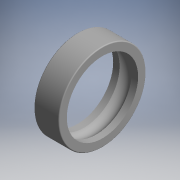
# Autodesk Inventor part: 6001JRX Outer Ring
Saved by Autodesk Inventor 2017.3 (Build 213256000, 256)
## iProperties
Part Number: 6001JRX Outer Ring
Material: Generic
Catalog Web Link: www.cadenas.de
Description: Open type or-Deep Groove Ball Bearings
Vendor: NTN
Document SubType Name: Modeling
Designer: partserver
Manufacturer: NTN
Mass: 1.44189 g
Surface Area: 17.2678 cm^2
Volume: 1.44189 cm^3
Density: 1 g/cm^3
Appearance: PSOLRGB-192-192-192
Category: PARTsolutions
Company: NTN
Title: 6001JRX Outer Ring
Author: Cadenas PARTsolutions
Comments: Deep Groove Ball Bearings
PSOL_IDENT_0: {$CADENAS_DATA\23d-libs\ntn\ball_roller_bearings\deep_groove_bb\deep_groove_bb\6_types\dgbb_or.prj},
PSOL_IDENT_1: 184 {VTYP=3D},{NB=6001JRX Outer Ring},{LINA=6001JRX Outer Ring},{NN=Open type or},{DATE=12.08.2020 0
PSOL_IDENT_2: 2:23:39},{GEOMDATE=13.03.2020 06:48:21},{VERSION=},{LINEID=8980},{WBVAR=},{WBNUMERIC=}  {NB=6001JRX
PSOL_IDENT_3: Outer Ring},{LINA=6001JRX Outer Ring},{KT=DUMMY},{IDNR=},{SD=12},{D=28},{B=8},{R=0.3},{ORDER1=6001JR
PSOL_IDENT_4: X},{ORDER=6001JRX},{NEWORDER=6001JRX},{CR=5.65},{COR=2.39},{CRF=MIN},{CORF=MIN},{LSG=26000},{LSO=300
PSOL_IDENT_5: 00},{MASS=0.021},{RNS=MIN},{LLH=MIN},{LLU=MIN},{ST=},{NCST=},{LTST=},{CST=},{SRG=},{SR=},{D1=26.44},
PSOL_IDENT_6: {A=2.20},{BA=0.90},{R0=0.30},{D2=MIN},{F=MIN},{DA1=},{DA2=},{DA=},{DX=MIN},{CY=},{CZ=},{RAS=},{RNAS=
PSOL_IDENT_7: 0.182},{VERS=1},{X=8},{N=7},{RB=2.40000},{O=62.80000}
NB: 6001JRX Outer Ring
NN: Open type or
NT: Deep Groove Ball Bearings
NBSYN: $ORDER. Outer Ring
LINA: 6001JRX Outer Ring
CATALOG: NTN Corporation
SD: 12
D: 28
B: 8
R: 0.3
ORDER1: 6001JRX
ORDER: 6001JRX
NEWORDER: 6001JRX
CR: 5.65
COR: 2.39
CRF: 0
CORF: 0
LSG: 26000
LSO: 30000
MASS: 0.021
RNS: 0
LLH: 0
LLU: 0
D1: 26.44
A: 2.2
BA: 0.9
R0: 0.3
D2: 0
F: 0
DX: 0
RNAS: 0.182
VERS: 1
SUPPLIER: NTN
ARTICLENO: 6001JRX Outer Ring
BOMINFO: 6001JRX Outer Ring
CREATOR: CADENAS GmbH
Autodesk Inventor part; units mm, degrees
sketch "Sketch_1" plane through (0, 0, 0) normal (0, 0, 1) x (1, 0, 0)
  line L0 (8, 0) -> (0, 0)
  line L1 (0, 11.44) -> (2.08, 11.44)
  arc A0 (5.92, 11.44) -> (2.08, 11.44) centre (4, 10) ccw
  line L2 (5.92, 11.44) -> (8, 11.44)
  line L3 (8, 11.44) -> (8, 13.7)
  arc A1 (8, 13.7) -> (7.7, 14) centre (7.7, 13.7) ccw
  line L4 (7.7, 14) -> (0.3, 14)
  arc A2 (0.3, 14) -> (0, 13.7) centre (0.3, 13.7) ccw
  line L5 (0, 13.7) -> (0, 11.44)
  constraints: 12 end point, 6 point on circle, 3 centre point
revolve "Revolution1" add sketch "Sketch_1" angle 360 about axis through (8, 0, 0) along (1, 0, 0)
ref_plane "dgbb_or_XY" through (0, 0, 0) normal (1, 0, 0) x (0, 0, -1)
ref_plane "dgbb_or_YZ" through (0, 0, 0) normal (0, 0, -1) x (0, 1, 0)
ref_plane "dgbb_or_ZX" through (0, 0, 0) normal (0, 1, 0) x (1, 0, 0)
ref_plane "dgbb_or1_XY" through (8, 0, 0) normal (1, 0, 0) x (0, 0, -1)
ref_plane "dgbb_or1_YZ" through (8, 0, 0) normal (0, 0, -1) x (0, 1, 0)
ref_plane "dgbb_or1_ZX" through (8, 0, 0) normal (0, 1, 0) x (1, 0, 0)
ref_plane "dgbb_or11_1_XY" through (4, 10, 0) normal (1, 0, 0) x (0, 0, -1)
ref_plane "dgbb_or11_1_YZ" through (4, 10, 0) normal (0, 0, -1) x (0, 1, 0)
ref_plane "dgbb_or11_1_ZX" through (4, 10, 0) normal (0, 1, 0) x (1, 0, 0)
ref_plane "dgbb_or11_2_XY" through (4, 6.2349, 7.8183) normal (1, 0, 0) x (0, 0, -1)
ref_plane "dgbb_or11_2_YZ" through (4, 6.2349, 7.8183) normal (0, 0, -1) x (0, 1, 0)
ref_plane "dgbb_or11_2_ZX" through (4, 6.2349, 7.8183) normal (0, 1, 0) x (1, 0, 0)
ref_plane "dgbb_or11_3_XY" through (4, -2.2252, 9.7493) normal (1, 0, 0) x (0, 0, -1)
ref_plane "dgbb_or11_3_YZ" through (4, -2.2252, 9.7493) normal (0, 0, -1) x (0, 1, 0)
ref_plane "dgbb_or11_3_ZX" through (4, -2.2252, 9.7493) normal (0, 1, 0) x (1, 0, 0)
ref_plane "dgbb_or11_4_XY" through (4, -9.0097, 4.3388) normal (1, 0, 0) x (0, 0, -1)
ref_plane "dgbb_or11_4_YZ" through (4, -9.0097, 4.3388) normal (0, 0, -1) x (0, 1, 0)
ref_plane "dgbb_or11_4_ZX" through (4, -9.0097, 4.3388) normal (0, 1, 0) x (1, 0, 0)
ref_plane "dgbb_or11_5_XY" through (4, -9.0097, -4.3388) normal (1, 0, 0) x (0, 0, -1)
ref_plane "dgbb_or11_5_YZ" through (4, -9.0097, -4.3388) normal (0, 0, -1) x (0, 1, 0)
ref_plane "dgbb_or11_5_ZX" through (4, -9.0097, -4.3388) normal (0, 1, 0) x (1, 0, 0)
ref_plane "dgbb_or11_6_XY" through (4, -2.2252, -9.7493) normal (1, 0, 0) x (0, 0, -1)
ref_plane "dgbb_or11_6_YZ" through (4, -2.2252, -9.7493) normal (0, 0, -1) x (0, 1, 0)
ref_plane "dgbb_or11_6_ZX" through (4, -2.2252, -9.7493) normal (0, 1, 0) x (1, 0, 0)
ref_plane "dgbb_or11_7_XY" through (4, 6.2349, -7.8183) normal (1, 0, 0) x (0, 0, -1)
ref_plane "dgbb_or11_7_YZ" through (4, 6.2349, -7.8183) normal (0, 0, -1) x (0, 1, 0)
ref_plane "dgbb_or11_7_ZX" through (4, 6.2349, -7.8183) normal (0, 1, 0) x (1, 0, 0)
body "Solid1"
